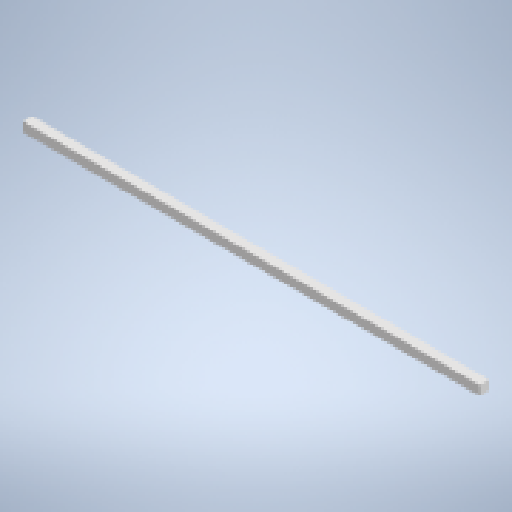
# Autodesk Inventor part: BarraMarco2.2
Saved by Autodesk Inventor 2024 (Build 280153000, 153)
## iProperties
Created: 2023-07-05
Part Number: BarraMarco2.2
Material: Genérico
Document SubType Name: Modeling
Designer: sergi
Density: 1 g/cm^3
Appearance: Valor por defecto
Author: sergi
Autodesk Inventor part; units mm, degrees
ref_plane "YZ Plane" through (0, 0, 0) normal (1, 0, 0) x (0, 1, 0)
ref_plane "XZ Plane" through (0, 0, 0) normal (0, 1, 0) x (-1, 0, 0)
ref_plane "XY Plane" through (0, 0, 0) normal (0, 0, 1) x (1, 0, 0)
sketch "Boceto1" plane through (0, 0, 0) normal (0, 0, 1) x (1, 0, 0)
  line L0 (-706.5, 15) -> (-706.5, 1360) projected
  line L1 (-706.5, 1360) -> (-185.5, 1360) projected
  line L2 (-185.5, 1360) -> (-185.5, 15) projected
  line L3 (-185.5, 15) -> (-706.5, 15) projected
  line L4 (692.5, -15) -> (692.5, -536) projected
  line L5 (692.5, -536) -> (-706.5, -536) projected
  line L6 (-706.5, -536) -> (-706.5, -15) projected
  line L7 (-706.5, -15) -> (692.5, -15) projected
  line L8 (722.5, -566) -> (722.5, 15) projected
  line L9 (722.5, 15) -> (-155.5, 15) projected
  line L10 (-155.5, 15) -> (-155.5, 1390) projected
  line L11 (-155.5, 1390) -> (-736.5, 1390) projected
  line L12 (-736.5, 1390) -> (-736.5, -566) projected
  line L13 (-736.5, -566) -> (722.5, -566) projected
  line L14 (692.5, -15) -> (722.5, -15)
  line L15 (-706.5, -15) -> (-736.5, -15)
  line L16 (-155.5, 15) -> (-185.5, 15)
  line L17 (-706.5, 15) -> (-736.5, 15)
  point P0 (0, 0)
  constraints: 8 end point, 6 point on line, 1 horizontal
extrude "Extrusión1" add sketch "Boceto1" against normal blind 30 contours L3 L16 L9 L8 L14 L7 L15 L12 L17
